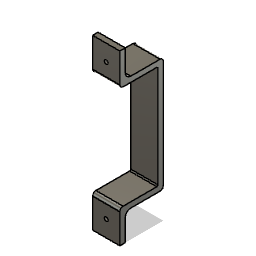
soportefuente (Autodesk Fusion 360 design; units mm, degrees)
Autodesk Fusion 360 part; units mm, degrees
sketch "Boceto1" plane through (0, 0, 0) normal (0, 1, 0) x (1, 0, 0)
sketch "Boceto2" plane through (0, 0, 0) normal (0, 0, 1) x (1, 0, 0)
  line L0 (0, 0) -> (0, 90)
  line L1 (0, 90) -> (25, 90)
  line L2 (0, 0) -> (25, 0)
  line L3 (25, 0) -> (25, 90)
  line L4 (25, 90) -> (25, 92)
  line L5 (25, 90) -> (25, 105)
  line L6 (25, 105) -> (0, 105)
  line L7 (0, 105) -> (0, 90)
  dimension "d1" = 90
  dimension "d2" = 25
  dimension "d4" = 15
  constraint coincident L0.start L2.start
  constraint vertical L0
  constraint perpendicular L0 L1
  constraint perpendicular L0 L2
  constraint perpendicular L1 L3
  constraint perpendicular L1 L4
  constraint perpendicular L1 L5
  constraint perpendicular L5 L6
  constraint perpendicular L1 L7
  measures "d1" distance of L0.start L0.end
  measures "d2" distance of L0.end L1.end
  measures "d4" distance of L1.end L5.end
extrude "Extruir1" add sketch "Boceto2" along normal blind 5
sketch "Boceto3" plane through (0, 0, 5) normal (0, 0, 1) x (1, 0, 0)
  line L0 (0, 0) -> (25, 0)
  line L1 (25, 0) -> (25, 105)
  line L2 (25, 105) -> (0, 105)
  line L3 (0, 105) -> (0, 0)
  line L4 (0, 0) -> (25, 0)
  line L5 (25, 0) -> (25, 5)
  line L6 (25, 5) -> (0, 5)
  line L7 (0, 5) -> (0, 0)
  line L8 (0, 105) -> (25, 105)
  line L9 (25, 105) -> (25, 100)
  line L10 (25, 100) -> (0, 100)
  line L11 (0, 100) -> (0, 105)
  dimension "d7" = 5
  dimension "d8" = 5
  constraint horizontal L4
  constraint vertical L5
  constraint horizontal L6
  constraint vertical L7
  constraint coincident L0.start L3.end
  constraint horizontal L8
  constraint vertical L9
  constraint horizontal L10
  constraint vertical L11
  constraint coincident L2.end L3.start
  measures "d7" distance of L0.start L6.end
  measures "d8" distance of L2.end L10.end
extrude "Extruir2" add sketch "Boceto3" along normal blind 35 contours L0 L1 L3 L4 L5 L6 L7 | L1 L2 L3 L8 L9 L10 L11
sketch "Boceto4" plane through (0, 0, 0) normal (0, 1, 0) x (1, 0, 0)
  line L0 (0, -40) -> (25, -40)
  line L1 (25, -40) -> (25, -35)
  line L2 (25, -35) -> (0, -35)
  line L3 (0, -35) -> (0, -40)
  dimension "d11" = 5
  constraint horizontal L0
  constraint vertical L1
  constraint horizontal L2
  constraint vertical L3
  measures "d11" distance of L0.start L2.end
extrude "Extruir3" add sketch "Boceto4" against normal blind 25
sketch "Boceto5" plane through (0, 105, 0) normal (0, 1, 0) x (-1, 0, 0)
  line L0 (-25, 0) -> (0, 0)
  line L1 (0, 0) -> (0, 40)
  line L2 (0, 40) -> (-25, 40)
  line L3 (-25, 40) -> (-25, 0)
  line L4 (-25, 40) -> (0, 40)
  line L5 (0, 40) -> (0, 35)
  line L6 (0, 35) -> (-25, 35)
  line L7 (-25, 35) -> (-25, 40)
  constraint horizontal L4
  constraint vertical L5
  constraint horizontal L6
  constraint vertical L7
  constraint coincident L1 L5.end
  constraint coincident L2.end L3.start
extrude "Extruir4" add sketch "Boceto5" along normal blind 25 contours L1 L2 L3 L4 L5 L6 L7
sketch "Boceto6" plane through (0, 0, 40) normal (0, 0, 1) x (1, 0, 0)
  line L0 (0, 100) -> (25, 100)
  line L1 (25, 100) -> (25, 130)
  line L2 (25, 130) -> (0, 130)
  line L3 (0, 130) -> (0, 100)
  line L4 (12.5, 130) -> (12.5, 115)
  circle A0 centre (12.5, 115) radius 1.75
  line L5 (0, 50) -> (30, 50)
  line L6 (0, -25) -> (25, -25)
  line L7 (12.5, -25) -> (12.5, -10)
  circle A1 centre (12.5, -10) radius 1.75
  dimension "d16" = 3.5
  dimension "d17" = 3.5
  constraint midpoint L2 L4.start
  constraint perpendicular L2 L4
  constraint coincident L4.end A0.centre
  constraint horizontal L5
  constraint horizontal L6
  constraint midpoint L6 L7.start
  constraint perpendicular L6 L7
  constraint coincident L7.end A1.centre
  measures "d16" diameter of A0
  measures "d17" diameter of A1
extrude "Extruir5" cut sketch "Boceto6" against normal blind 5 contours A0 | A1
fillet "Empalme1" radius 5 1 edges at (12.5, 105, 35)
fillet "Empalme2" radius 5 1 edges at (12.5, 0, 35)
fillet "Empalme3" radius 3 4 edges at (12.5, 0, 0) (12.5, 105, 0) (12.5, 100, 40) (12.5, 5, 40)
fillet "Empalme4" radius 1 2 edges at (12.5, 5, 5) (12.5, 100, 5)
